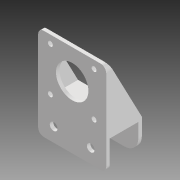
# Autodesk Inventor part: MotorBracket1
Saved by Autodesk Inventor 2020 (Build 240168000, 168)
## iProperties
Created: 2020-10-22
Part Number: MotorBracket1
Material: Generic
Document SubType Name: Modeling
Designer: DDeGo
Density: 1 g/cm^3
Appearance: Default
Author: DDeGo
Autodesk Inventor part; units mm, degrees
ref_plane "YZ Plane" through (0, 0, 0) normal (1, 0, 0) x (0, 1, 0)
ref_plane "XZ Plane" through (0, 0, 0) normal (0, 1, 0) x (-1, 0, 0)
ref_plane "XY Plane" through (0, 0, 0) normal (0, 0, 1) x (1, 0, 0)
sketch "Sketch1" plane through (0, 0, 0) normal (0, 0, 1) x (1, 0, 0)
  line L0 (-21.15, -21.15) -> (21.15, -21.15) construction
  line L1 (21.15, -21.15) -> (21.15, 21.15)
  line L2 (21.15, 21.15) -> (-21.15, 21.15)
  line L3 (-21.15, 21.15) -> (-21.15, -21.15)
  line L4 (-21.15, -21.15) -> (21.15, 21.15) construction
  line L5 (21.15, -21.15) -> (-21.15, 21.15) construction
  line L6 (15.5, 15.5) -> (-15.5, 15.5) construction
  line L7 (-15.5, 15.5) -> (-15.5, -15.5) construction
  line L8 (-15.5, -15.5) -> (15.5, -15.5) construction
  line L9 (15.5, -15.5) -> (15.5, 15.5) construction
  line L10 (15.5, 15.5) -> (-15.5, -15.5) construction
  line L11 (-15.5, 15.5) -> (15.5, -15.5) construction
  line L12 (-21.15, -21.15) -> (-21.15, -44.15)
  line L13 (-21.15, -44.15) -> (21.15, -44.15)
  line L14 (21.15, -44.15) -> (21.15, -21.15)
  line L15 (21.15, -34.15) -> (-21.15, -34.15) construction
  circle A0 centre (-13.15, -34.15) radius 2.75
  circle A1 centre (13.15, -34.15) radius 2.75
  circle A2 centre (0, 0) radius 11.5
  circle A3 centre (-15.5, -15.5) radius 1.75
  circle A4 centre (15.5, -15.5) radius 1.75
  circle A5 centre (-15.5, 15.5) radius 1.75
  circle A6 centre (15.5, 15.5) radius 1.75
  dimension "d0" = 42.3
  dimension "d1" = 42.3
  dimension "d2" = 10
  dimension "d3" = 23
  dimension "d4" = 8
  dimension "d5" = 8
  dimension "d6" = 5.5
  dimension "d7" = 31
  dimension "d8" = 3.5
  dimension "d9" = 23
  constraints: 32 end point, 7 centre point, 5 coincident, 5 perpendicular, 5 point on line, 4 equal radius, 4 midpoint, 4 parallel, 2 horizontal, 1 vertical
  measures "d0" distance of L1.end L2.end
  measures "d1" distance of L0.end L1.end
  measures "d2" distance between parallel lines of L13 L15
  measures "d3" distance between parallel lines of L0 L13
  measures "d4" distance from line of L14 A1.centre
  measures "d5" distance from line of L12 A0.centre
  measures "d6" diameter of A0
  measures "d7" distance of L7.end L8.end
  measures "d8" diameter of A5
  measures "d9" diameter of A2
extrude "Extrusion1" add sketch "Sketch1" along normal blind 2.5
sketch "Sketch2" plane through (21.15, -44.15, 0) normal (1, 0, 0) x (0, 0, -1)
  line L0 (0, 0) -> (-2.5, 0) construction
  line L1 (0, 65.3) -> (-2.5, 65.3) construction
  line L2 (-2.5, 0) -> (-2.5, 65.3) construction
  line L3 (-2.5, 65.3) -> (0, 65.3) construction
  line L4 (0, 65.3) -> (20.3, 22) construction
  line L5 (20.3, 22) -> (20.3, 0)
  line L6 (20.3, 0) -> (-2.5, 0) construction
  line L7 (20.3, 22) -> (0, 22)
  line L8 (0, 22) -> (0, 65.3)
  line L9 (20.3, 0) -> (22.8, 0)
  line L10 (22.8, 0) -> (22.8, 22)
  line L11 (0, 0) -> (0, 65.3) projected
  line L12 (22.8, 22) -> (0, 65.3)
  line L13 (20.3, 22) -> (22.8, 22) construction
  line L14 (0, 0) -> (0, 65.3) projected
  line L15 (0, 65.3) -> (-2.5, 65.3) projected
  line L16 (-2.5, 0) -> (-2.5, 65.3) projected
  line L17 (0, 0) -> (-2.5, 0) projected
  point P0 (0, 44.15)
  point P1 (0, 65.3)
  dimension "d12" = 22
  dimension "d14" = 2.5
  dimension "d28" = 20.3
  constraints: 22 end point, 5 perpendicular, 3 horizontal, 1 parallel
  measures "d12" distance of L4.end L5.end
  measures "d14" distance of L4.end L10.end
  measures "d28" distance between parallel lines of L5 L14
extrude "Extrusion2" add sketch "Sketch2" along normal blind 3
mirror "Mirror1" about plane through (0, 0, 0) normal (1, 0, 0) of "Extrusion2"
sketch "Sketch3" plane through (-21.15, -44.15, -20.3) normal (1, 0, 0) x (0, 0, -1)
  line L0 (0, 22) -> (0, 0) projected
  line L1 (0, 22) -> (2.5, 22)
  line L2 (2.5, 22) -> (2.5, 0)
  line L3 (2.5, 0) -> (0, 0)
  line L4 (0, 0) -> (0, 22)
  point P0 (-20.3, 44.15)
  constraints: 8 end point, 2 parallel, 1 horizontal, 1 perpendicular
extrude "Extrusion3" add sketch "Sketch3" along normal up to surface (42.3 mm away)
sketch "Sketch4" plane through (24.15, -44.15, -20.3) normal (0, 0, 1) x (1, 0, 0)
  line L0 (-45.3, 22) -> (-48.3, 22) projected
  line L1 (0, 22) -> (0, 0) projected
  line L2 (-48.3, 22) -> (0, 22)
  line L3 (0, 22) -> (0, 20)
  line L4 (0, 20) -> (-48.3, 20)
  line L5 (-48.3, 20) -> (-48.3, 22)
  point P0 (-24.15, 44.15)
  point P1 (0, 22)
  dimension "d19" = 2
  constraints: 8 end point, 2 parallel, 1 horizontal, 1 perpendicular, 1 point on line
  measures "d19" distance between parallel lines of L4 L2
extrude "Extrusion4" add sketch "Sketch4" along normal up to surface (20.3 mm away)
sketch "Sketch5" plane through (24.15, -44.15, -22.8) normal (0, 0, -1) x (-1, 0, 0)
  line L0 (48.3, 0) -> (0, 0) projected
  line L1 (24.15, 0) -> (24.15, 10) construction
  circle A0 centre (24.15, 10) radius 2.75
  point P0 (24.15, 44.15)
  dimension "d22" = 5.5
  dimension "d23" = 10
  constraints: 2 end point, 1 centre point, 1 coincident, 1 midpoint, 1 vertical
  measures "d22" diameter of A0
  measures "d23" distance of L1.start L1.end
extrude "Extrusion5" cut sketch "Sketch5" against normal up to surface (2.5 mm away)
fillet "Fillet1" radius 10 2 edges at (24.15, -44.15, -21.55) (-24.15, -44.15, -21.55)
fillet "Fillet1" radius 4 4 edges at (-24.15, -44.15, 1.25) (24.15, -44.15, 1.25) (24.15, 21.15, 1.25) (-24.15, 21.15, 1.25)
body "Solid1"
